Autodesk Fusion 360 part; units mm, degrees
(part 2 of 2)
  constraint tangent L213 A234
  constraint tangent L214 A234
  constraint tangent L214 A235
  constraint tangent L215 A235
  constraint tangent L215 A236
  constraint tangent L216 A236
  constraint tangent L216 A237
  constraint tangent L217 A237
  constraint tangent L218 A238
  constraint tangent L219 A238
  constraint tangent L217 A239
  constraint tangent L218 A239
  constraint tangent L220 A240
  constraint tangent L221 A240
  constraint tangent L219 A241
  constraint tangent L220 A241
  constraint coincident L106.end L200
  constraint perpendicular L106 L200
  constraint horizontal L230
  constraint coincident L199 L230.end
  constraint perpendicular L199 L231
  constraint coincident L199 L232.start
  constraint perpendicular L222 L232
  constraint coincident L222 L232.end
  constraint parallel L237 L238
  constraint parallel L243 L244
  constraint tangent L239 A242
  constraint tangent L243 A242
  constraint tangent L240 A243
  constraint tangent L243 A243
  constraint tangent L241 A244
  constraint tangent L244 A244
  constraint tangent L242 A245
  constraint tangent L244 A245
  constraint tangent L234 A246
  constraint tangent L237 A246
  constraint tangent L233 A247
  constraint tangent L237 A247
  constraint tangent L236 A248
  constraint tangent L238 A248
  constraint tangent L235 A249
  constraint tangent L238 A249
  constraint parallel L249 L250
  constraint tangent L247 A250
  constraint tangent L249 A250
  constraint tangent L248 A251
  constraint tangent L249 A251
  constraint tangent L245 A252
  constraint tangent L250 A252
  constraint tangent L246 A253
  constraint tangent L250 A253
  constraint parallel L255 L256
  constraint tangent L253 A254
  constraint tangent L255 A254
  constraint tangent L254 A255
  constraint tangent L255 A255
  constraint tangent L251 A256
  constraint tangent L256 A256
  constraint tangent L252 A257
  constraint tangent L256 A257
  constraint tangent L107 A258
  constraint tangent L108 A258
  constraint tangent L108 A259
  constraint tangent L230 A259
  constraint tangent L106 A260
  constraint tangent L107 A260
  constraint tangent L110 A261
  constraint tangent L231 A261
  constraint tangent L109 A262
  constraint tangent L110 A262
  measures "d1" diameter of A0
  measures "d2" diameter of A1
  measures "d3" diameter of A2
  measures "d4" diameter of A3
  measures "d5" diameter of A4
  measures "d9" diameter of A111
  measures "d12" diameter of A112
extrude "Extrude1" add sketch "mriya" along normal blind 10.6 contours L185 A198 L186 A199 L187 A200 L188 A201 L189 A202 L190 A203 L191 A204 L192 A205 L193 A206 L194 A207 L195 A208 L196 A209 L197 A210 L198 A211 L199 L200 A213 L201 A214 L202 A215 L203 A216 L204 A217 L205 A218 L206 A219 L207 L208 L209 A220 L210 A221 L211 L212 L213 L214 L215 L216 L217 L218 L219 L220 L221 L222 A223 L223 L224 L225 L226 L227 L228 A224 A225 A226 A227 A228 A229 A230 A231 L229 A232 A233 A234 A235 A236 A237 A238 A239 A240 A241 L232 picked at (-141.416666, 51.759867) makes body 1
extrude "Extrude2" add sketch "mriya" along normal blind 17.1 contours L199 A212 L200 L221 A222 L222 L229 L232 picked at (-5.283334, 44.5932) bodies 1
extrude "Extrude3" add sketch "mriya" along normal blind 2 from surface at 1.7 contours L106 L107 L108 L109 L110 L185 A198 L186 A199 L187 A200 L188 A201 L189 A202 L190 A203 L191 A204 L192 A205 L193 A206 L194 A207 L195 A208 L196 A209 L197 A210 L198 A211 L199 L200 A213 L201 A214 L202 A215 L203 A216 L204 A217 L205 A218 L206 A219 L230 L231 A258 A259 A260 A261 A262 | L106 L107 L108 L199 A212 L200 L230 A258 A259 A260 | L109 L110 L199 L231 A261 A262 | A114 | A115 | A116 | A117 picked at (-84.826309, 24.168075) picked at (-7.216667, 50.959867) picked at (-7.216666, 8.059867) picked at (-64.728451, 82.79316) picked at (-45.728484, 78.29313) picked at (-25.071567, 2.493271) picked at (-44.071558, 4.793248) bodies 1
extrude "Extrude6" add sketch "mriya" along normal blind 1 from surface at 14.3 contours L106 L107 L108 L199 A212 L200 L230 A258 A259 A260 picked at (-7.216667, 50.959867) bodies 1
extrude "Extrude7" add sketch "mriya" along normal blind 1 from surface at 7.8 contours L109 L110 L199 L231 A261 A262 picked at (-7.216666, 8.059867) bodies 1
sketch "power-switch" plane through (-4.449999, 0, 0) normal (1, 0, 0) x (0, 1, 0)
  line L0 (19.1932, 0) -> (76.4932, 0)
  line L1 (76.4932, 0) -> (76.4932, 16.8)
  line L2 (76.4932, 16.8) -> (19.1932, 16.8)
  line L3 (19.1932, 16.8) -> (19.1932, 10.5)
  line L4 (36.0932, 5.1) -> (25.6932, 5.1)
  line L5 (25.6932, 5.1) -> (25.6932, 8)
  line L6 (25.6932, 8) -> (36.0932, 8)
  line L7 (36.0932, 8) -> (36.0932, 5.1)
  line L8 (37.4932, 3.6) -> (24.2932, 3.6)
  line L9 (23.8932, 4) -> (23.8932, 9.1)
  line L10 (24.2932, 9.5) -> (37.4932, 9.5)
  line L11 (37.8932, 9.1) -> (37.8932, 4)
  line L12 (19.1932, 10.5) -> (19.1932, 0)
  line L13 (1.9932, 0) -> (76.4932, 0)
  line L14 (76.4932, 0) -> (76.4932, 17.1)
  line L15 (76.4932, 17.1) -> (19.2932, 17.1)
  line L16 (19.2932, 17.1) -> (19.2932, 10.6)
  line L17 (19.2932, 10.6) -> (1.9932, 10.6)
  line L18 (1.9932, 10.6) -> (1.9932, 0)
  arc A0 (37.8932, 9.1) -> (37.4932, 9.5) centre (37.4932, 9.1) ccw
  arc A1 (37.4932, 3.6) -> (37.8932, 4) centre (37.4932, 4) ccw
  arc A2 (23.8932, 4) -> (24.2932, 3.6) centre (24.2932, 4) ccw
  arc A3 (24.2932, 9.5) -> (23.8932, 9.1) centre (24.2932, 9.1) ccw
  constraint perpendicular L4 L5
  constraint vertical L5
  constraint perpendicular L5 L6
  constraint vertical L7
  constraint tangent L10 A0
  constraint tangent L11 A0
  constraint tangent L11 A1
  constraint tangent L8 A1
  constraint tangent L8 A2
  constraint tangent L9 A2
  constraint tangent L9 A3
  constraint tangent L10 A3
extrude "Extrude8" cut sketch "power-switch" against normal blind 2.5 contours L4 L5 L6 L7 picked at (32.626533, 6.066667) bodies 1
extrude "Extrude9" cut sketch "power-switch" against normal blind 1 contours L8 L9 L10 L11 A0 A1 A2 A3 picked at (24.4932, 7.033333) bodies 1
chamfer "Chamfer5" distance 0.8 angle 45 4 edges at (-6.949999, 30.8932, 5.1) (-6.949999, 36.0932, 6.55) (-6.949999, 30.8932, 8) (-6.949999, 25.6932, 6.55) on bodies 1
chamfer "Chamfer9" distance 1 angle 45 8 edges at (-4.449999, 30.8932, 3.6) (-4.45, 24.010357, 3.717157) (-4.449999, 23.8932, 6.55) (-4.45, 24.010357, 9.382843) (-4.449999, 30.8932, 9.5) (-4.45, 37.776043, 9.382843) (-4.449999, 37.8932, 6.55) (-4.45, 37.776043, 3.717157) on bodies 1
sketch "usb-c" plane through (0, 80.6432, 0) normal (0, 1, 0) x (-1, 0, 0)
  line L0 (3.6, 0) -> (36.129542, 0)
  line L1 (3.6, 16.7) -> (3.6, 0)
  line L2 (21.20025, 10.9) -> (21.20025, 10.1)
  arc A0 (21.20025, 10.9) -> (19.80025, 12.3) centre (19.80025, 10.9) ccw
  line L3 (11.80025, 10.1) -> (11.80025, 10.9)
  line L4 (19.80025, 8.7) -> (13.20025, 8.7)
  line L5 (21.20025, 7.3) -> (11.80025, 7.3)
  arc A1 (11.80025, 10.1) -> (13.20025, 8.7) centre (13.20025, 10.1) ccw
  line L6 (22.20025, 12.7) -> (22.20025, 8.3)
  line L7 (11.80025, 13.7) -> (21.20025, 13.7)
  arc A2 (13.20025, 12.3) -> (11.80025, 10.9) centre (13.20025, 10.9) ccw
  arc A3 (19.80025, 8.7) -> (21.20025, 10.1) centre (19.80025, 10.1) ccw
  line L8 (10.80025, 8.3) -> (10.80025, 12.7)
  line L9 (13.20025, 12.3) -> (19.80025, 12.3)
  line L10 (8.600001, 0) -> (25.9, 0)
  line L11 (25.9, 10.5) -> (25.9, 16.8)
  line L12 (25.9, 16.8) -> (8.600001, 16.8)
  line L13 (8.600001, 16.8) -> (8.600001, 0)
  line L14 (25.9, 0) -> (25.9, 10.5)
  line L15 (8.600001, 0) -> (41.088119, 0)
  line L16 (41.088119, 0) -> (41.088119, 10.5)
  line L17 (41.088119, 10.5) -> (25.9, 10.5)
  line L18 (25.9, 10.5) -> (25.9, 17)
  line L19 (25.9, 17) -> (8.600001, 17)
  line L20 (8.600001, 17) -> (8.600001, 0)
  line L21 (8.600001, 0) -> (41.088119, 0)
  line L22 (41.088119, 0) -> (41.088119, 10.6)
  line L23 (41.088119, 10.6) -> (25.8, 10.6)
  line L24 (25.8, 10.6) -> (25.8, 17.1)
  line L25 (25.8, 17.1) -> (8.600001, 17.1)
  line L26 (8.600001, 17.1) -> (8.600001, 0)
  arc A4 (11.80025, 13.7) -> (10.80025, 12.7) centre (11.80025, 12.7) ccw
  arc A5 (22.20025, 12.7) -> (21.20025, 13.7) centre (21.20025, 12.7) ccw
  arc A6 (10.80025, 8.3) -> (11.80025, 7.3) centre (11.80025, 8.3) ccw
  arc A7 (21.20025, 7.3) -> (22.20025, 8.3) centre (21.20025, 8.3) ccw
  constraint tangent L3 A2
  constraint tangent A2 L9
  constraint tangent A0 L9
  constraint tangent L2 A0
  constraint tangent L4 A3
  constraint tangent L2 A3
  constraint tangent L4 A1
  constraint tangent L3 A1
  constraint perpendicular L6 L7
  constraint perpendicular L5 L8
  constraint horizontal L5
  constraint perpendicular L5 L6
  constraint tangent L8 A4
  constraint tangent L7 A4
  constraint tangent L7 A5
  constraint tangent L6 A5
  constraint tangent L5 A6
  constraint tangent L8 A6
  constraint tangent L6 A7
  constraint tangent L5 A7
extrude "Extrude10" cut sketch "usb-c" against normal blind 2.5 contours L2 A0 L3 L4 A1 A2 A3 L9 picked at (15.40025, 11.1) bodies 1
extrude "Extrude11" cut sketch "usb-c" against normal blind 1 contours L5 L6 L7 L8 A4 A5 A6 A7 picked at (15.40025, 13.233333) bodies 1
chamfer "Chamfer10" distance 1 angle 45 8 edges at (-10.80025, 80.6432, 10.5) (-11.093143, 80.6432, 13.407107) (-16.50025, 80.6432, 13.7) (-21.907357, 80.6432, 13.407107) (-22.20025, 80.6432, 10.5) (-21.907357, 80.6432, 7.592893) (-16.50025, 80.6432, 7.3) (-11.093143, 80.6432, 7.592893) on bodies 1
chamfer "Chamfer11" distance 0.79 angle 45 4 edges at (-6.950001, 57.2432, 14.3) (-7.433275, 77.659926, 14.3) (-14.850001, 78.1432, 14.3) (-6.95, 9.5932, 7.8) on bodies 1
chamfer "Chamfer4" distance 1 angle 45 90 edges at (-33.44406, 80.6432, 10.6) (-41.470803, 80.71932, 10.6) (-42.359441, 81.500307, 10.6) (-43.896925, 82.71484, 10.6) (-51.46655, 82.943201, 10.6) (-58.272149, 83.019604, 10.6) (-60.260642, 84.900676, 10.6) (-62.896988, 87.214745, 10.6) (-73.400145, 87.443199, 10.6) (-83.903077, 87.214838, 10.6) (-86.040561, 85.400306, 10.6) (-87.529198, 84.019319, 10.6) (-94.833454, 83.943199, 10.6) (-102.903076, 83.714837, 10.6) (-107.217336, 79.723529, 10.6) (-111.044961, 76.05738, 10.6) (-116.187006, 75.9432, 10.6) (-121.903076, 75.714838, 10.6) (-123.440559, 74.500307, 10.6) (-124.329196, 73.71932, 10.6) (-131.40594, 73.6432, 10.6) (-141.034493, 72.427693, 10.6) (-142.25, 42.8932, 10.6) (-141.034493, 13.358707, 10.6) (-120.382982, 12.1432, 10.6) (-100.94415, 12.485634, 10.6) (-96.434572, 16.509865, 10.6) (-92.737435, 19.99135, 10.6) (-84.585569, 20.143201, 10.6) (-75.68512, 19.734247, 10.6) (-70.518243, 11.420229, 10.6) (-65.168056, 2.920317, 10.6) (-56.057903, 2.443204, 10.6) (-48.329196, 2.367084, 10.6) (-47.440558, 1.586096, 10.6) (-45.903073, 0.371562, 10.6) (-37.233452, 0.143202, 10.6) (-29.34028, 0.069542, 10.6) (-28.450122, -0.712016, 10.6) (-26.904053, -1.929959, 10.6) (-17.179837, -2.156801, 10.6) (-5.665506, -0.941293, 10.6) (-4.45, 10.6432, 10.6) (-17.200001, 80.6432, 17.1) (-4.450001, 47.8932, 17.1) (-5.665508, 79.427693, 17.1) (-4.45, 39.2432, 0) (-5.665508, 79.427693, 0) (-24.84406, 80.6432, 0) (-41.470803, 80.71932, 0) (-42.359441, 81.500307, 0) (-43.896925, 82.71484, 0) (-51.46655, 82.943201, 0) (-58.272149, 83.019604, 0) (-60.260642, 84.900676, 0) (-62.896988, 87.214745, 0) (-73.400145, 87.443199, 0) (-83.903077, 87.214838, 0) (-86.040561, 85.400306, 0) (-87.529198, 84.019319, 0) (-94.833454, 83.943199, 0) (-102.903076, 83.714837, 0) (-107.217336, 79.723529, 0) (-111.044961, 76.05738, 0) (-116.187006, 75.9432, 0) (-121.903076, 75.714838, 0) (-123.440559, 74.500307, 0) (-124.329196, 73.71932, 0) (-131.40594, 73.6432, 0) (-141.034493, 72.427693, 0) (-142.25, 42.8932, 0) (-141.034493, 13.358707, 0) (-120.382982, 12.1432, 0) (-100.94415, 12.485634, 0) (-96.434572, 16.509865, 0) (-92.737435, 19.99135, 0) (-84.585569, 20.143201, 0) (-75.68512, 19.734247, 0) (-70.518243, 11.420229, 0) (-65.168056, 2.920317, 0) (-56.057903, 2.443204, 0) (-48.329196, 2.367084, 0) (-47.440558, 1.586096, 0) (-45.903073, 0.371562, 0) (-37.233452, 0.143202, 0) (-29.34028, 0.069542, 0) (-28.450122, -0.712016, 0) (-26.904053, -1.929959, 0) (-17.179837, -2.156801, 0) (-5.665506, -0.941293, 0) on bodies 1
fillet "Fillet27" radius 1.2 1 edges at (-4.45, 19.2932, 12.85) on bodies 1
chamfer "Chamfer6" distance 1 angle 45 2 edges at (-6.3, 19.2932, 17.1) (-5.549648, 19.297403, 17.1) on bodies 1
mirror "Mirror1" about plane through (0, 0, 0) normal (1, 0, 0) of bodies 1 makes body 2
named bodies: "Left", "Right"
